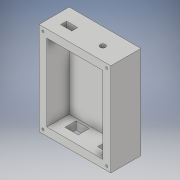
# Autodesk Inventor part: arduinoCase
Saved by Autodesk Inventor 2017 (Build 210142000, 142)
## iProperties
Created: 2017-04-16
Part Number: arduinoCase
Material: Generic
Document SubType Name: Modeling
Designer: rocke
Density: 1 g/cm^3
Appearance: Default
Author: rocke
Autodesk Inventor part; units mm, degrees
ref_plane "YZ Plane" through (0, 0, 0) normal (1, 0, 0) x (0, 1, 0)
ref_plane "XZ Plane" through (0, 0, 0) normal (0, 1, 0) x (-1, 0, 0)
ref_plane "XY Plane" through (0, 0, 0) normal (0, 0, 1) x (1, 0, 0)
sketch "Sketch8" plane through (0, 0, 0) normal (0, 0, 1) x (1, 0, 0)
  line L0 (0, 0) -> (68.834, 0)
  line L1 (68.834, 0) -> (68.834, 89.027)
  line L2 (68.834, 89.027) -> (0, 89.027)
  line L3 (0, 89.027) -> (0, 0)
  dimension "d20" = 89.027
  dimension "d21" = 68.834
  constraints: 8 end point, 2 parallel, 1 horizontal, 1 perpendicular
  measures "d20" distance of L0.end L1.end
  measures "d21" distance of L1.end L2.end
extrude "Extrusion6" add sketch "Sketch8" along normal blind 28.956
shell "Shell2" thickness 7.62 removed faces 1 at (45.8893, 29.6757, 28.956)
sketch "Sketch9" plane through (0, 0, 0) normal (0, -1, 0) x (1, 0, 0)
  point P0 (0, 0)
sketch "Sketch10" plane through (0, 0, 0) normal (0, -1, 0) x (1, 0, 0)
  line L0 (16.51, 20.5994) -> (29.21, 20.5994)
  line L1 (29.21, 20.5994) -> (29.21, 9.9314)
  line L2 (29.21, 9.9314) -> (16.51, 9.9314)
  line L3 (16.51, 9.9314) -> (16.51, 20.5994)
  line L4 (0, 0) -> (68.834, 0) projected
  line L5 (0, 0) -> (0, 28.956) projected
  line L6 (48.26, 20.9296) -> (57.15, 20.9296)
  line L7 (57.15, 20.9296) -> (57.15, 9.9314)
  line L8 (57.15, 9.9314) -> (48.26, 9.9314)
  line L9 (48.26, 9.9314) -> (48.26, 20.9296)
  line L10 (68.834, 0) -> (68.834, 28.956) projected
  dimension "d25" = 10.668
  dimension "d26" = 12.7
  dimension "d27" = 9.9314
  dimension "d28" = 16.51
  dimension "d29" = 10.9982
  dimension "d30" = 8.89
  dimension "d31" = 9.9314
  dimension "d32" = 11.684
  constraints: 16 end point, 4 parallel, 2 horizontal, 2 perpendicular
  measures "d25" distance of L0.end L1.end
  measures "d26" distance of L1.end L2.end
  measures "d27" distance between parallel lines of L4 L2
  measures "d28" distance between parallel lines of L5 L3
  measures "d29" distance of L6.end L7.end
  measures "d30" distance of L7.end L8.end
  measures "d31" distance between parallel lines of L4 L8
  measures "d32" distance between parallel lines of L10 L7
extrude "Extrusion7" cut sketch "Sketch10" against normal blind 28.956 contours L0 L1 L2 L3
extrude "Extrusion8" cut sketch "Sketch10" against normal blind 28.956 contours L6 L7 L8 L9
sketch "Sketch11" plane through (7.62, 81.407, 7.62) normal (0, -1, 0) x (1, 0, 0)
  point P0 (-7.62, -7.62)
sketch "Sketch12" plane through (0, 89.027, 0) normal (0, 1, 0) x (1, 0, 0)
  circle A0 centre (48.514, -16.256) radius 2.5
  line L0 (68.834, 0) -> (68.834, -28.956) projected
  line L1 (68.834, -28.956) -> (0, -28.956) projected
  point P0 (0, 0)
  dimension "d37" = 5
  dimension "d38" = 20.32
  dimension "d39" = 12.7
  constraints: 1 centre point
  measures "d37" diameter of A0
  measures "d38" distance from line of L0 A0.centre
  measures "d39" distance from line of L1 A0.centre
extrude "Extrusion9" cut sketch "Sketch12" against normal blind 28.956
sketch "Sketch13" plane through (0, 0, 28.956) normal (0, 0, 1) x (1, 0, 0)
  line L0 (0, 89.027) -> (0, 0) projected
  line L1 (0, 89.027) -> (7.62, 81.407)
  circle A0 centre (3.81, 85.217) radius 1.0414
  line L2 (7.62, 81.407) -> (61.214, 81.407) projected
  line L3 (61.214, 81.407) -> (68.834, 89.027)
  line L4 (7.62, 7.62) -> (61.214, 7.62) projected
  line L5 (7.62, 7.62) -> (0, 0)
  line L6 (0, 0) -> (68.834, 0) projected
  line L7 (61.214, 7.62) -> (68.834, 0)
  circle A1 centre (65.024, 85.217) radius 1.0414
  circle A2 centre (3.81, 3.81) radius 1.0414
  circle A3 centre (65.024, 3.81) radius 1.0414
  dimension "d42" = 2.0828
  dimension "d43" = 2.0828
  dimension "d44" = 2.0828
  dimension "d45" = 2.0828
  constraints: 8 end point, 4 centre point, 4 midpoint
  measures "d42" diameter of A0
  measures "d43" diameter of A1
  measures "d44" diameter of A2
  measures "d45" diameter of A3
extrude "Extrusion10" cut sketch "Sketch13" against normal blind 17.78 contours A0 L1 | L1 A0
extrude "Extrusion11" cut sketch "Sketch13" against normal blind 17.78 contours A1 L3 | L3 A1
extrude "Extrusion12" cut sketch "Sketch13" against normal blind 17.78 contours A2 L5 | L5 A2
extrude "Extrusion13" cut sketch "Sketch13" against normal blind 17.78 contours A3 L7 | L7 A3
sketch "Sketch14" plane through (0, 89.027, 0) normal (0, 1, 0) x (1, 0, 0)
  line L0 (21.2173, -18.756) -> (10.5493, -18.756)
  line L1 (10.5493, -18.756) -> (10.5493, -13.168)
  line L2 (10.5493, -13.168) -> (21.2173, -13.168)
  line L3 (21.2173, -13.168) -> (21.2173, -18.756)
  circle A0 centre (48.514, -16.256) radius 2.5 projected
  point P0 (0, 0)
  dimension "d54" = 10.668
  dimension "d55" = 5.588
  dimension "d56" = 0
  constraints: 8 end point, 2 parallel, 1 horizontal, 1 perpendicular
  measures "d54" distance of L1.end L2.end
  measures "d55" distance of L0.end L1.end
  measures "d56" distance edge to line of A0 L0
extrude "Extrusion14" cut sketch "Sketch14" against normal blind 17.78 contours L0 L1 L2 L3
body "Solid2"
